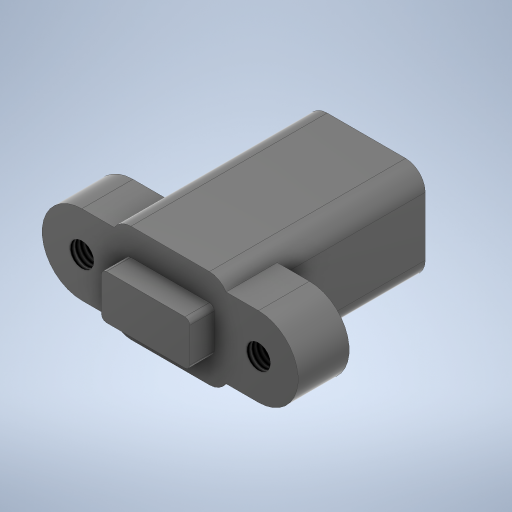
# Autodesk Inventor part: 103367_Panel_Side_USB
Saved by Autodesk Inventor 2023 (Build 270158000, 158)
## iProperties
Created: 2023-09-26
Part Number: 103367_Panel_Side_USB
Material: Generic
Document SubType Name: Modeling
Designer: Graeme
Density: 1 g/cm^3
Appearance: Default
Author: Graeme
Autodesk Inventor part; units mm, degrees
ref_plane "YZ Plane" through (0, 0, 0) normal (1, 0, 0) x (0, 1, 0)
ref_plane "XZ Plane" through (0, 0, 0) normal (0, 1, 0) x (-1, 0, 0)
ref_plane "XY Plane" through (0, 0, 0) normal (0, 0, 1) x (1, 0, 0)
sketch "Sketch1" plane through (0, 0, 0) normal (0, 0, 1) x (1, 0, 0)
  line L0 (-4.5, -2.26) -> (4.5, -2.26)
  line L1 (4.5, -2.26) -> (4.5, 2.26)
  line L2 (4.5, 2.26) -> (-4.5, 2.26)
  line L3 (-4.5, 2.26) -> (-4.5, -2.26)
  line L4 (-4.5, -2.26) -> (4.5, 2.26) construction
  line L5 (4.5, -2.26) -> (-4.5, 2.26) construction
  point P0 (0, 0)
  dimension "d0" = 9
  dimension "d1" = 4.52
  constraints: 12 end point, 2 midpoint, 2 parallel, 1 horizontal, 1 perpendicular
  measures "d0" distance of L2.end L1.end
  measures "d1" distance of L1.end L0.end
extrude "Extrusion1" add sketch "Sketch1" along normal blind 2.5
sketch "Sketch2" plane through (0, 0, 0) normal (0, 0, 1) x (1, 0, 0)
  line L0 (-6, -5) -> (6, -5)
  line L1 (6, -5) -> (6, 5)
  line L2 (6, 5) -> (-6, 5)
  line L3 (-6, 5) -> (-6, -5)
  line L4 (-6, -5) -> (6, 5) construction
  line L5 (6, -5) -> (-6, 5) construction
  point P0 (0, 0)
  dimension "d4" = 12
  dimension "d5" = 10
  constraints: 12 end point, 2 midpoint, 2 parallel, 1 horizontal, 1 perpendicular
  measures "d4" distance of L2.end L1.end
  measures "d5" distance of L1.end L0.end
extrude "Extrusion2" add sketch "Sketch2" against normal blind 20
fillet "Fillet1" radius 2 4 edges at (-6, 5, -10) (6, 5, -10) (6, -5, -10) (-6, -5, -10)
sketch "Sketch3" plane through (0, 0, 0) normal (0, 0, 1) x (1, 0, 0)
  line L0 (-9, 0) -> (9, 0) construction
  circle A0 centre (-9, 0) radius 4.05
  circle A1 centre (9, 0) radius 4.05
  line L1 (-9, 4.05) -> (9, 4.05)
  line L2 (9, 4.05) -> (9, -4.05)
  line L3 (9, -4.05) -> (-9, -4.05)
  line L4 (-9, -4.05) -> (-9, 4.05)
  point P0 (0, 0)
  point P1 (0, 0)
  dimension "d10" = 8.1
  dimension "d9" = 18
  constraints: 10 end point, 5 coincident, 2 horizontal, 2 midpoint, 2 parallel, 1 perpendicular, 6 other
  measures "d9" distance of L0.end L0.start
extrude "Extrusion3" add sketch "Sketch3" against normal blind 5.2
hole "Hole1" at (-9, 0, 0) at (9, 0, 0) direction (0, 0, -1) diameter 2.459 end through all thread size "M3x0.5" class "6H" standard "ISO Metric profile"
fillet "Fillet2" radius 0.5 4 edges at (-4.5, 2.26, 1.25) (4.5, 2.26, 1.25) (4.5, -2.26, 1.25) (-4.5, -2.26, 1.25)
body "Solid1"
